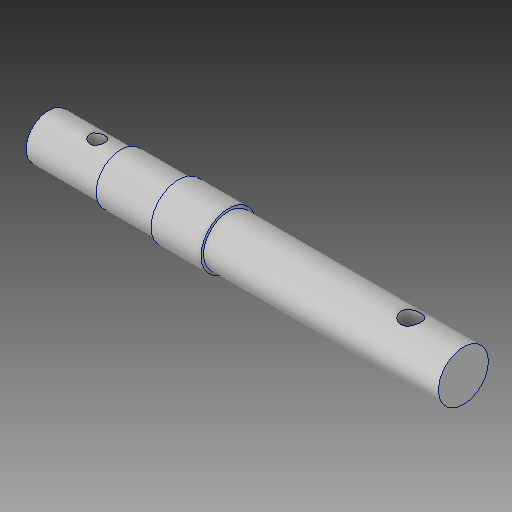
# Autodesk Inventor part: Shaft_main
Saved by Autodesk Inventor 2018 (Build 220112000, 112)
## iProperties
Created: 2017-10-20
Part Number: Shaft_main
Material: アルミニウム 6061
Document SubType Name: Modeling
Designer: 翔
Density: 2.7 g/cm^3
Appearance: アルミニウム - フラット
Author: 翔
Autodesk Inventor part; units mm, degrees
ref_plane "YZ Plane" through (0, 0, 0) normal (1, 0, 0) x (0, 1, 0)
ref_plane "XY Plane" through (0, 0, 0) normal (0, 0, 1) x (1, 0, 0)
sketch "スケッチ1" plane through (0, 0, 0) normal (0, 1, 0) x (-1, 0, 0)
  line L0 (199.2, 0) -> (-33.2, 0) projected
  line L1 (0, -13.2) -> (0, 2.2) projected
  line L2 (166, 0) -> (166, -9)
  line L3 (114, -11) -> (94, -11)
  line L4 (94, -11) -> (94, -10)
  line L5 (94, -10) -> (0, -10)
  line L6 (0, -10) -> (0, 0)
  line L7 (166, 0) -> (0, 0)
  line L8 (166, -9) -> (137, -9)
  line L9 (137, -9) -> (137, -10)
  line L10 (137, -10) -> (114, -10)
  line L11 (114, -10) -> (114, -11)
  dimension "d1" = 11
  dimension "d2" = 10
  dimension "d3" = 9
  dimension "d4" = 10
  dimension "d6" = 29
  dimension "d8" = 23
  dimension "d9" = 20
  dimension "d10" = 166
  constraints: 20 end point, 6 perpendicular, 2 collinear, 1 point on line
  measures "d1" distance between parallel lines of L0 L3
  measures "d2" distance between parallel lines of L0 L10
  measures "d3" distance between parallel lines of L0 L8
  measures "d4" distance between parallel lines of L0 L5
  measures "d6" distance between parallel lines of L9 L2
  measures "d8" distance between parallel lines of L11 L9
  measures "d9" distance between parallel lines of L4 L11
  measures "d10" distance between parallel lines of L6 L2
revolve "回転1" add sketch "スケッチ1" angle 360 about axis through (-166, 0, 0) along (1, 0, 0)
sketch "スケッチ2" plane through (0, 0, 0) normal (0, 1, 0) x (-1, 0, 0)
  circle A0 centre (21, 0) radius 4
  line L0 (0, 10) -> (0, -10) projected
  point P0 (0, 0)
  dimension "d12" = 8
  dimension "d13" = 21
  constraints: 1 centre point
  measures "d12" diameter of A0
  measures "d13" distance from line of L0 A0.centre
extrude "押し出し2" cut sketch "スケッチ2" along normal through all both and the other way through all
ref_plane "作業平面1" through (0, 9, 0) normal (0, 1, 0) x (-1, 0, 0)
sketch "スケッチ3" plane through (0, 9, 0) normal (0, 1, 0) x (-1, 0, 0)
  line L0 (166, 9) -> (166, -9) projected
  point P0 (0, 0)
  point P1 (146.5, 0)
  dimension "d19" = 19.5
  measures "d19" distance from line of point (146.5, 0) L0
hole "穴1" at (-146.5, 9, 0) direction (0, -1, 0) diameter 6 depth 8 tip angle 118
